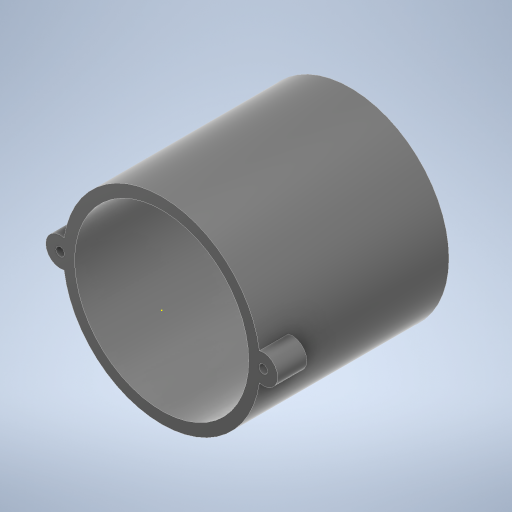
# Autodesk Inventor part: osłonasilnik
Saved by Autodesk Inventor 2024 (Build 280153000, 153)
## iProperties
Created: 2025-05-23
Part Number: osłonasilnik
Material: Tworzywo sztuczne PET
Document SubType Name: Modeling
Designer: Paweł
Density: 1.541 g/cm^3
Appearance: Gładki — czarny
Mass: 81.8908 g
Surface Area: 282.864 cm^2
Volume: 53.1414 cm^3
Author: Paweł
Autodesk Inventor part; units mm, degrees
ref_plane "YZ Plane" through (0, 0, 0) normal (1, 0, 0) x (0, 1, 0)
ref_plane "XZ Plane" through (0, 0, 0) normal (0, 1, 0) x (-1, 0, 0)
ref_plane "XY Plane" through (0, 0, 0) normal (0, 0, 1) x (1, 0, 0)
sketch "Szkic1" plane through (0, 0, 0) normal (0, 0, 1) x (1, 0, 0)
  circle A0 centre (0, 0) radius 30
  circle A1 centre (0, 0) radius 34
  dimension "d0" = 60
  dimension "d1" = 4
  constraints: 2 centre point, 1 coincident
  measures "d0" diameter of A0
  measures "d1" radial gap between concentric circles of A0 A1
extrude "Wyciągnięcie proste1" add sketch "Szkic1" along normal blind 65
sketch "Szkic2" plane through (0, 0, 65) normal (0, 0, 1) x (1, 0, 0)
  circle A0 centre (35, 0) radius 5
  circle A1 centre (0, 0) radius 34 projected
  circle A2 centre (0, 0) radius 30 projected
  circle A3 centre (35, 0) radius 1.5
  line L0 (0, 0) -> (0, -30)
  circle A4 centre (-35, 0) radius 5
  circle A5 centre (-35, 0) radius 1.5
  point P0 (33.9821, 1.1018)
  point P1 (33.9821, -1.1018)
  point P2 (33.6571, -4.8163)
  point P3 (33.6571, 4.8163)
  point P4 (-33.9821, -1.1018)
  point P5 (-33.9821, 1.1018)
  point P6 (-33.6571, 4.8163)
  point P7 (-33.6571, -4.8163)
  dimension "d5" = 10
  dimension "d6" = 3
  dimension "d9" = 70
  constraints: 4 centre point, 2 coincident, 2 end point, 2 symmetric about line, 1 vertical, 1 vertical alignment, 4 other
  measures "d5" diameter of A0
  measures "d6" diameter of A3
  measures "d9" distance of A4.centre A0.centre
extrude "Wyciągnięcie proste2" add sketch "Szkic2" against normal blind 10 contours A0 A1 A3 | A1 A5 A4 picked at (35.0063, -3.323) picked at (-35.0802, 3.3077)
sketch "Szkic3" plane through (0, 0, 65) normal (0, 0, 1) x (1, 0, 0)
  point P0 (0, 0)
sketch "Szkic4" plane through (0, 0, 65) normal (0, 0, 1) x (1, 0, 0)
  arc A0 (-33.9821, 1.1018) -> (-33.9821, -1.1018) centre (-35, 0) ccw projected
  circle A1 centre (-35, 0) radius 1.5
  arc A2 (33.9821, -1.1018) -> (33.9821, 1.1018) centre (35, 0) ccw projected
  circle A3 centre (35, 0) radius 1.5
  point P0 (0, 0)
  point P1 (33.9821, 1.1018)
  point P2 (33.9821, -1.1018)
  point P3 (-33.9821, -1.1018)
  point P4 (-33.9821, 1.1018)
  constraints: 2 centre point, 2 coincident
extrude "Wyciągnięcie proste3" cut sketch "Szkic4" against normal blind 10
